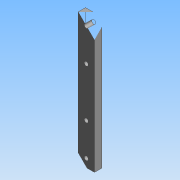
# Autodesk Inventor part: holdersupport
Saved by Autodesk Inventor 2015 (Build 190159000, 159)
## iProperties
Created: 2014-09-02
Part Number: holdersupport
Material: Generic
Document SubType Name: Modeling
Designer: shohei
Density: 1 g/cm^3
Appearance: Default
Author: shohei
Autodesk Inventor part; units mm, degrees
ref_plane "YZ Plane" through (0, 0, 0) normal (1, 0, 0) x (0, 1, 0)
ref_plane "XZ Plane" through (0, 0, 0) normal (0, 1, 0) x (-1, 0, 0)
ref_plane "XY Plane" through (0, 0, 0) normal (0, 0, 1) x (1, 0, 0)
sketch "Sketch4" plane through (0, 0, 0) normal (0, 1, 0) x (-1, 0, 0)
  line L0 (0, 0) -> (20, 0)
  line L1 (20, 0) -> (20, 120)
  line L2 (20, 120) -> (0, 120)
  line L3 (0, 120) -> (0, 0)
  circle A0 centre (10, 10) radius 2.5
  circle A1 centre (10, 110) radius 2.5
  circle A2 centre (10, 70) radius 2.5
  line L4 (0, 0) -> (20, 0)
  line L5 (20, 0) -> (20, -40)
  line L6 (20, -40) -> (0, -40)
  line L7 (0, -40) -> (0, 0)
  circle A3 centre (10, -30) radius 2.5
  dimension "d0" = 120
  dimension "d3" = 20
  dimension "d4" = 5
  dimension "d5" = 10
  dimension "d6" = 10
  dimension "d7" = 5
  dimension "d8" = 10
  dimension "d9" = 10
  dimension "d12" = 5
  dimension "d13" = 60
  dimension "d16" = 40
  dimension "d17" = 5
  dimension "d18" = 10
  dimension "d19" = 10
  constraints: 16 end point, 4 centre point, 4 parallel, 2 horizontal, 2 perpendicular
  measures "d0" distance of L0.end L1.end
  measures "d3" distance of L1.end L2.end
  measures "d4" diameter of A0
  measures "d5" distance from line of L1 A0.centre
  measures "d6" distance from line of L0 A0.centre
  measures "d7" diameter of A1
  measures "d8" distance from line of L3 A1.centre
  measures "d9" distance from line of L2 A1.centre
  measures "d12" diameter of A2
  measures "d13" distance of A0.centre A2.centre
  measures "d16" distance of L4.end L5.end
  measures "d17" diameter of A3
  measures "d18" distance from line of L7 A3.centre
  measures "d19" distance from line of L6 A3.centre
extrude "Extrusion3" add sketch "Sketch4" along normal blind 9 contours L3 L2 L1 L0
sketch "Sketch5" plane through (0, 9, 0) normal (0, 1, 0) x (1, 0, 0)
  line L0 (60, -20) -> (-20, -20) projected
  circle A0 centre (-10, -10) radius 2.5 projected
  circle A1 centre (50, -10) radius 2.5 projected
  line L1 (-20, -20) -> (-20, 0) projected
  line L2 (60, -20) -> (-20, -20) projected
  line L3 (60, 0) -> (60, -20) projected
  line L4 (-20, 0) -> (60, 0) projected
  circle A2 centre (-10, -70) radius 2.5 projected
  circle A3 centre (-10, -110) radius 2.5 projected
  circle A4 centre (-10, -10) radius 2.5 projected
  line L5 (0, 0) -> (-20, 0) projected
  line L6 (-20, 0) -> (-20, -120) projected
  line L7 (-20, -120) -> (0, -120) projected
  line L8 (0, -120) -> (0, 0) projected
  line L9 (-20, 0) -> (0, 0)
  line L10 (0, 0) -> (0, 40)
  line L11 (0, 40) -> (-20, 40)
  line L12 (-20, 40) -> (-20, 0)
  circle A5 centre (-10, 30) radius 2.5
  dimension "d20" = 40
  dimension "d21" = 5
  dimension "d22" = 10
  dimension "d23" = 10
  constraints: 8 end point, 2 parallel, 1 centre point, 1 horizontal, 1 perpendicular
  measures "d20" distance of L11.end L5.end
  measures "d21" diameter of A5
  measures "d22" distance from line of L10 A5.centre
  measures "d23" distance from line of L11 A5.centre
extrude "Extrusion4" add sketch "Sketch5" against normal blind 9 contours L4 L12 L11 L10
body "Solid3"
